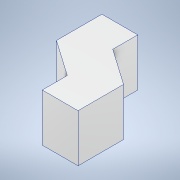
# Autodesk Inventor part: Soporte Riel
Saved by Autodesk Inventor 2020.3 (Build 243373000, 373)
## iProperties
Created: 2020-07-21
Part Number: Soporte Riel
Material: Aluminum 6061
Document SubType Name: Modeling
Designer: juanp
Density: 2.7 g/cm^3
Appearance: Aluminum - Flat
Author: juanp
Autodesk Inventor part; units mm, degrees
ref_plane "YZ Plane" through (0, 0, 0) normal (1, 0, 0) x (0, 1, 0)
ref_plane "XZ Plane" through (0, 0, 0) normal (0, 1, 0) x (-1, 0, 0)
ref_plane "XY Plane" through (0, 0, 0) normal (0, 0, 1) x (1, 0, 0)
sketch "Sketch1" plane through (0, 0, 0) normal (0, 1, 0) x (-1, 0, 0)
  line L0 (0, 0) -> (0, -19.05)
  line L1 (30, -20.95) -> (30, -40)
  line L2 (0, 0) -> (30, -20.95) construction
  line L3 (0, -19.05) -> (30, -40) construction
  line L4 (15, 0) -> (0, 0)
  line L5 (15, 0) -> (15, -50) construction
  line L6 (15, 0) -> (15, -10.475)
  line L7 (15, -10.475) -> (30, -20.95)
  line L8 (30, -40) -> (15, -40)
  line L9 (15, -29.525) -> (15, -40)
  line L10 (15, -29.525) -> (0, -19.05)
  line L11 (0, 0) -> (30, 0) construction
  point P0 (15, 0)
  dimension "d0" = 19.05
  dimension "d1" = 19.05
  dimension "d2" = 30
  dimension "d3" = 20.95
  dimension "d4" = 50
  dimension "d5" = 30
  constraints: 24 end point, 4 point on line, 3 collinear, 3 midpoint, 2 horizontal, 2 perpendicular, 2 vertical
  measures "d0" distance of L0.start L0.end
  measures "d1" distance of L1.start L1.end
  measures "d2" distance between parallel lines of L0 L1
  measures "d3" vertical distance of L1.end L0.end
  measures "d4" distance of L4.start L5.end
  measures "d5" distance of L0.start L11.end
extrude "Extrusion1" add sketch "Sketch1" along normal blind 20
body "Solid1"
